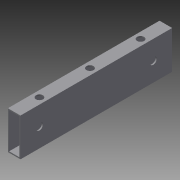
# Autodesk Inventor part: 090000-1
Saved by Autodesk Inventor 2015 (Build 190159000, 159)
## iProperties
Created: 2015-05-09
Part Number: 090000-1
Material: Generic
Document SubType Name: Modeling
Designer: Wesley
Density: 1 g/cm^3
Appearance: Default
Author: Wesley
Autodesk Inventor part; units mm, degrees
ref_plane "YZ Plane" through (0, 0, 0) normal (1, 0, 0) x (0, 1, 0)
ref_plane "XZ Plane" through (0, 0, 0) normal (0, 1, 0) x (-1, 0, 0)
ref_plane "XY Plane" through (0, 0, 0) normal (0, 0, 1) x (1, 0, 0)
sketch "Sketch1" plane through (0, 0, 0) normal (0, 0, 1) x (1, 0, 0)
  line L0 (0, 0) -> (12.7, 0)
  line L1 (12.7, 0) -> (12.7, 38.1)
  line L2 (12.7, 38.1) -> (0, 38.1)
  line L3 (0, 38.1) -> (0, 0)
  dimension "d0" = 38.1
  dimension "d1" = 12.7
  constraints: 8 end point, 2 parallel, 1 horizontal, 1 perpendicular
  measures "d0" distance of L2.end L0.start
  measures "d1" distance of L0.start L0.end
extrude "Extrusion1" add sketch "Sketch1" along normal blind 152.4
shell "Shell1" thickness 1.27 removed faces 2 at (4.2333, 25.4, 0) at (4.2333, 25.4, 152.4)
sketch "Sketch2" plane through (12.7, 0, 0) normal (1, 0, 0) x (0, 0, -1)
  line L0 (0, 0) -> (0, 38.1) projected
  line L1 (0, 38.1) -> (-152.4, 38.1) projected
  line L2 (-152.4, 0) -> (-152.4, 38.1) projected
  line L3 (0, 0) -> (-152.4, 0) projected
  line L4 (-162.6393, 19.05) -> (14.976, 19.05) construction
  point P0 (-133.35, 19.05)
  point P1 (-19.05, 19.05)
  dimension "d5" = 19.05
  dimension "d6" = 19.05
  dimension "d9" = 19.05
  constraints: 2 end point, 2 point on line, 1 horizontal
  measures "d5" distance between parallel lines of L3 L4
  measures "d6" distance from line of L2 point (-133.35, 19.05)
  measures "d9" distance from line of L0 point (-19.05, 19.05)
hole "Hole1" at (12.7, 19.05, 133.35) at (12.7, 19.05, 19.05) direction (-1, 0, 0) diameter 7.112 end through all
sketch "Sketch3" plane through (0, 38.1, 0) normal (0, 1, 0) x (1, 0, 0)
  line L0 (12.7, 0) -> (0, 0) projected
  line L1 (0, 0) -> (0, -152.4) projected
  line L2 (12.7, -152.4) -> (0, -152.4) projected
  line L3 (12.7, 0) -> (12.7, -152.4) projected
  line L4 (6.35, 17.6784) -> (6.35, -171.0582) construction
  point P0 (0, 0)
  point P1 (6.35, -25.4)
  point P2 (6.35, -127)
  point P3 (6.35, -76.2)
  dimension "d17" = 6.35
  dimension "d18" = 25.4
  dimension "d19" = 25.4
  dimension "d20" = 76.2
  constraints: 3 point on line, 2 end point, 1 vertical
  measures "d17" distance between parallel lines of L1 L4
  measures "d18" distance from line of L0 point (6.35, -25.4)
  measures "d19" distance from line of L2 point (6.35, -127)
  measures "d20" distance from line of L0 point (6.35, -76.2)
hole "Hole2" at (6.35, 38.1, 25.4) at (6.35, 38.1, 127) at (6.35, 38.1, 76.2) direction (0, -1, 0) diameter 7.112 end through all
body "Solid1"
